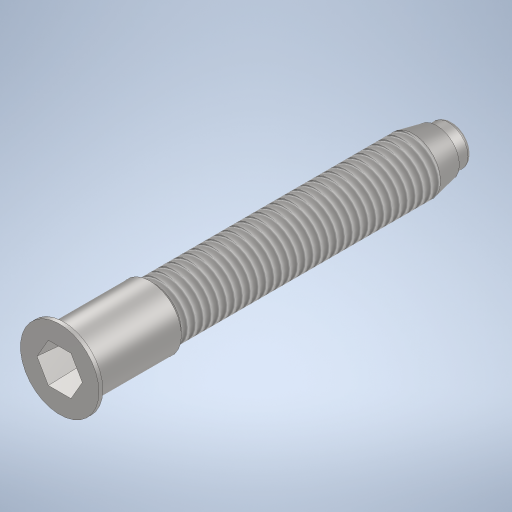
# Autodesk Inventor part: Confirmat Joint110100
Saved by Autodesk Inventor 2024 (Build 280153000, 153)
## iProperties
RuleStatus: InUse
Part Number: Confirmat Joint110100
Material: Generic
Document SubType Name: Modeling
Designer: RokasM
Density: 1 g/cm^3
Appearance: Default
Author: RokasM
Autodesk Inventor part; units mm, degrees
ref_plane "YZ Plane" through (0, 0, 0) normal (1, 0, 0) x (0, 1, 0)
ref_plane "XZ Plane" through (0, 0, 0) normal (0, 1, 0) x (-1, 0, 0)
ref_plane "XY Plane" through (0, 0, 0) normal (0, 0, 1) x (1, 0, 0)
sketch "Sketch1" plane through (0, 0, 0) normal (0, 0, 1) x (1, 0, 0)
  circle A0 centre (0, 0) radius 5
  dimension "d0" = 10
  constraints: 1 centre point, 1 coincident
  measures "d0" diameter of A0
extrude "Extrusion1" add sketch "Sketch1" against normal blind 1
chamfer "Chamfer1" distance 1 distance2 0.5 1 edges at (-5, 0, -1) measured on face at (-4.5, 0, -1)
sketch "Sketch2" plane through (0, 0, -1) normal (0, 0, -1) x (-1, 0, 0)
  circle A0 centre (0, 0) radius 4 projected
extrude "Extrusion2" add sketch "Sketch2" along normal blind 11
chamfer "Chamfer2" distance 0.5 angle 45 1 edges at (4, 0, -12)
sketch "Sketch3" plane through (0, 0, -12) normal (0, 0, -1) x (-1, 0, 0)
  circle A0 centre (0, 0) radius 3.5 projected
extrude "Extrusion3" add sketch "Sketch3" along normal blind 33
sketch "Sketch4" plane through (0, 0, -45) normal (0, 0, -1) x (-1, 0, 0)
  circle A0 centre (0, 0) radius 3.5 projected
extrude "Extrusion4" add sketch "Sketch4" along normal blind 3
chamfer "Chamfer3" distance 0.6 distance2 3 1 edges at (3.5, 0, -48) measured on face at (3, 0, -48)
sketch "Sketch5" plane through (0, 0, -48) normal (0, 0, -1) x (-1, 0, 0)
  circle A0 centre (0, 0) radius 2.9 projected
  circle A1 centre (0, 0) radius 2.5
  dimension "d18" = 0.4
  constraints: 1 centre point
  measures "d18" radial gap between concentric circles of A0 A1
extrude "Extrusion5" add sketch "Sketch5" along normal blind 2 contours A1
thread "Thread1" size "M7x1" class "6g" standard "ISO Metric profile" full length
fillet "Fillet1" radius 0.5 1 edges at (2.5, 0, -50)
sketch "Sketch6" plane through (0, 0, 0) normal (0, 0, 1) x (1, 0, 0)
  line L0 (1.4434, 2.5) -> (2.8868, 0)
  line L1 (2.8868, 0) -> (1.4434, -2.5)
  line L2 (1.4434, -2.5) -> (-1.4434, -2.5)
  line L3 (-1.4434, -2.5) -> (-2.8868, 0)
  line L4 (-2.8868, 0) -> (-1.4434, 2.5)
  line L5 (-1.4434, 2.5) -> (1.4434, 2.5)
  point P0 (0, 0)
  point P1 (0, 0)
  dimension "d22" = 5
  constraints: 12 end point, 1 coincident, 1 horizontal, 13 other
  measures "d22" distance between parallel lines of L2 L5
extrude "Extrusion6" cut sketch "Sketch6" against normal blind 4 draft -5
sketch "Sketch7" plane through (0, 0, 0) normal (0, 0, 1) x (1, 0, 0)
  circle A0 centre (0, 0) radius 4 projected
extrude "Extrusion7" add sketch "Sketch7" against normal blind 18 separate body
sketch "Sketch8" plane through (0, 0, -18) normal (0, 0, -1) x (-1, 0, 0)
  circle A0 centre (0, 0.061) radius 2.5
  point P0 (0, 0)
  dimension "d27" = 5
  constraints: 1 centre point
  measures "d27" diameter of A0
extrude "Extrusion8" add sketch "Sketch8" along normal blind 33 bodies 2
equation "\"d25\" = Nestled_Board_Thickness"
equation "\"Nestled_Board_Thickness\" = 18"
